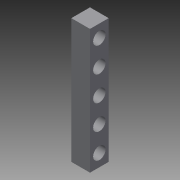
# Autodesk Inventor part: gripper_mc_dipper
Saved by Autodesk Inventor 2015 (Build 190159000, 159)
## iProperties
Created: 2015-01-15
Part Number: gripper_mc_dipper
Material: Generic
Document SubType Name: Modeling
Designer: Tucker
Density: 1 g/cm^3
Appearance: Default
Author: Tucker
Autodesk Inventor part; units mm, degrees
ref_plane "YZ Plane" through (0, 0, 0) normal (1, 0, 0) x (0, 1, 0)
ref_plane "XZ Plane" through (0, 0, 0) normal (0, 1, 0) x (-1, 0, 0)
ref_plane "XY Plane" through (0, 0, 0) normal (0, 0, 1) x (1, 0, 0)
sketch "Sketch2" plane through (0, 0, 0) normal (1, 0, 0) x (0, 1, 0)
  line L0 (0, 0) -> (508, 0)
  line L1 (508, 0) -> (508, -76.2)
  line L2 (508, -76.2) -> (0, -76.2)
  line L3 (0, -76.2) -> (0, 0)
  dimension "d0" = 508
  dimension "d1" = 76.2
  constraints: 8 end point, 2 parallel, 1 horizontal, 1 perpendicular
  measures "d0" distance of L1.end L2.end
  measures "d1" distance of L0.end L1.end
extrude "Extrusion1" add sketch "Sketch2" along normal blind 76.2
sketch "Sketch4" plane through (76.2, 0, 0) normal (1, 0, 0) x (0, 0, -1)
  circle A0 centre (38.1, 50.8) radius 25.4
  circle A1 centre (38.1, 152.4) radius 25.4
  circle A2 centre (38.1, 254) radius 25.4
  circle A3 centre (38.1, 355.6) radius 25.4
  circle A4 centre (38.1, 457.2) radius 25.4
  point P0 (0, 0)
  dimension "d10" = 50.8
  dimension "d11" = 50.8
  dimension "d12" = 50.8
  dimension "d13" = 50.8
  dimension "d14" = 50.8
  constraints: 5 centre point
  measures "d10" diameter of A0
  measures "d11" diameter of A1
  measures "d12" diameter of A2
  measures "d13" diameter of A3
  measures "d14" diameter of A4
extrude "Extrusion3" cut sketch "Sketch4" against normal blind 76.2
body "Solid1"
